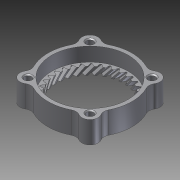
# Autodesk Inventor part: Inner_Helical_Gear_34.5mmOD_3x11.5mmID_4mmH_0.1mmBL_40deg_0.8mmM_33T_CCW_Nema17
Saved by Autodesk Inventor 2015 (Build 190159000, 159)
## iProperties
Created: 2014-08-15
Part Number: Inner_Helical_Gear_34.5mmOD_3x11.5mmID_4mmH_0.1mmBL_40deg_0.8mmM_33T_CCW_Nema17
Material: Generic
Document SubType Name: Modeling
Designer: User
Density: 1 g/cm^3
Appearance: Default
Author: User
Autodesk Inventor part; units mm, degrees
ref_plane "YZ Plane" through (0, 0, 0) normal (1, 0, 0) x (0, 1, 0)
ref_plane "XZ Plane" through (0, 0, 0) normal (0, 1, 0) x (-1, 0, 0)
ref_plane "XY Plane" through (0, 0, 0) normal (0, 0, 1) x (1, 0, 0)
sketch "Sketch1" plane through (0, 0, 0) normal (0, 0, 1) x (1, 0, 0)
  spline S0 degree 3 poles (-1.1058, 16.6253) (-1.0811, 16.7025) (-1.0316, 16.857) (-0.9463, 17.0848) (-0.8539, 17.3098) (-0.7542, 17.5317) (-0.6479, 17.7505) (-0.5354, 17.9662) (-0.4175, 18.1789) (-0.3342, 18.3181) (-0.2926, 18.3877) knots 0 0 0 0 0.124996 0.249995 0.374995 0.499995 0.624996 0.749997 0.874998 1 1 1 1
  spline S1 degree 3 poles (1.1058, 16.6253) (1.0811, 16.7025) (1.0316, 16.857) (0.9463, 17.0848) (0.8539, 17.3098) (0.7542, 17.5317) (0.6479, 17.7505) (0.5354, 17.9662) (0.4175, 18.1789) (0.3342, 18.3181) (0.2926, 18.3877) knots 0 0 0 0 0.124996 0.249995 0.374995 0.499995 0.624996 0.749997 0.874998 1 1 1 1
  circle A0 centre (0, 0) radius 18.39 construction
  circle A1 centre (0, 0) radius 15.5639 construction
  circle A2 centre (0, 0) radius 17.2314 construction
  circle A3 centre (0, 0) radius 16.6621
  circle A4 centre (0, 0) radius 20.118
  arc A5 (0.2926, 18.3877) -> (-0.2926, 18.3877) centre (0, 0) ccw
  point P0 (-1.0298, 16.8563)
  point P1 (-0.9451, 17.0843)
  point P2 (-0.8527, 17.3093)
  point P3 (-0.7531, 17.5312)
  point P4 (-0.6469, 17.75)
  point P5 (-0.5345, 17.9657)
  point P6 (-0.4163, 18.1783)
  point P7 (1.0298, 16.8563)
  point P8 (0.9451, 17.0843)
  point P9 (0.8527, 17.3093)
  point P10 (0.7531, 17.5312)
  point P11 (0.6469, 17.75)
  point P12 (0.5345, 17.9657)
  point P13 (0.4163, 18.1783)
  constraints: 6 centre point, 6 point on circle, 43 other
extrude "Extrusion1" add sketch "Sketch1" against normal blind 4 contours S0 A5 S1 A3 | A4
coil "Coil1" sketch "Sketch1" operation cut axis through (0, 0, -10) along (0, 0, -1) pitch 129.0296 turns 0.031001 hand left contours S0 A5 S1 A3
pattern_circular "Circular Pattern1" count 33 over 360 about axis through (0, 0, 0) along (0, 0, -1) of "Coil1"
sketch "Sketch2" plane through (0, 0, 0) normal (0, 0, 1) x (1, 0, 0)
  line L0 (-15.5, 15.5) -> (15.5, 15.5) construction
  line L1 (15.5, 15.5) -> (15.5, -15.5) construction
  line L2 (15.5, -15.5) -> (-15.5, -15.5) construction
  line L3 (-15.5, -15.5) -> (-15.5, 15.5) construction
  arc A0 (18.9021, 13.3963) -> (13.3963, 18.9021) centre (15.5, 15.5) ccw
  arc A1 (13.3963, -18.9021) -> (18.9021, -13.3963) centre (15.5, -15.5) ccw
  arc A2 (-18.9021, -13.3963) -> (-13.3963, -18.9021) centre (-15.5, -15.5) ccw
  arc A3 (-13.3963, 18.9021) -> (-18.9021, 13.3963) centre (-15.5, 15.5) ccw
  arc A4 (18.7355, -9.4857) -> (18.7355, 9.4857) centre (0, 0) ccw
  arc A5 (-9.4857, -18.7355) -> (9.4857, -18.7355) centre (0, 0) ccw
  arc A6 (9.4857, 18.7355) -> (-9.4857, 18.7355) centre (0, 0) ccw
  arc A7 (-18.7355, 9.4857) -> (-18.7355, -9.4857) centre (0, 0) ccw
  arc A8 (-13.3963, 18.9021) -> (-9.4857, 18.7355) centre (-11.2926, 22.3042) ccw
  arc A9 (9.4857, 18.7355) -> (13.3963, 18.9021) centre (11.2926, 22.3042) ccw
  arc A10 (18.9021, 13.3963) -> (18.7355, 9.4857) centre (22.3042, 11.2926) ccw
  arc A11 (18.7355, -9.4857) -> (18.9021, -13.3963) centre (22.3042, -11.2926) ccw
  arc A12 (13.3963, -18.9021) -> (9.4857, -18.7355) centre (11.2926, -22.3042) ccw
  arc A13 (-9.4857, -18.7355) -> (-13.3963, -18.9021) centre (-11.2926, -22.3042) ccw
  arc A14 (-18.9021, -13.3963) -> (-18.7355, -9.4857) centre (-22.3042, -11.2926) ccw
  arc A15 (-18.7355, 9.4857) -> (-18.9021, 13.3963) centre (-22.3042, 11.2926) ccw
  circle A16 centre (0, 0) radius 20.118 projected
  point P0 (15.5, 0)
  point P1 (0, 15.5)
  dimension "d14" = 31
  dimension "d15" = 31
  dimension "d16" = 8
  dimension "d17" = 8
  dimension "d18" = 8
  dimension "d19" = 8
  dimension "d20" = 21
  dimension "d21" = 21
  dimension "d22" = 21
  dimension "d23" = 21
  dimension "d24" = 4
  constraints: 32 point on circle, 16 centre point, 16 tangent, 8 end point, 7 equal radius, 5 coincident, 2 midpoint, 2 parallel, 1 horizontal, 1 horizontal alignment, 1 perpendicular, 1 vertical alignment
  measures "d14" distance of L0.start L0.end
  measures "d15" distance of L0.end L1.end
  measures "d16" diameter of A0
  measures "d17" diameter of A1
  measures "d18" diameter of A2
  measures "d19" diameter of A3
  measures "d20" radius of A4
  measures "d21" radius of A6
  measures "d22" radius of A7
  measures "d23" radius of A5
  measures "d24" radius of A8
extrude "Extrusion2" add sketch "Sketch2" against normal blind 4
sketch "Sketch3" plane through (0, 0, 0) normal (0, 0, 1) x (1, 0, 0)
  arc A0 (-13.3963, 18.9021) -> (-9.4857, 18.7355) centre (-11.2926, 22.3042) ccw projected
  arc A1 (-13.3963, 18.9021) -> (-18.9021, 13.3963) centre (-15.5, 15.5) ccw projected
  arc A2 (-18.7355, 9.4857) -> (-18.9021, 13.3963) centre (-22.3042, 11.2926) ccw projected
  arc A3 (-18.7355, 9.4857) -> (-18.7355, -9.4857) centre (0, 0) ccw projected
  arc A4 (-18.9021, -13.3963) -> (-18.7355, -9.4857) centre (-22.3042, -11.2926) ccw projected
  arc A5 (-18.9021, -13.3963) -> (-13.3963, -18.9021) centre (-15.5, -15.5) ccw projected
  arc A6 (-9.4857, -18.7355) -> (-13.3963, -18.9021) centre (-11.2926, -22.3042) ccw projected
  arc A7 (-9.4857, -18.7355) -> (9.4857, -18.7355) centre (0, 0) ccw projected
  arc A8 (13.3963, -18.9021) -> (9.4857, -18.7355) centre (11.2926, -22.3042) ccw projected
  arc A9 (13.3963, -18.9021) -> (18.9021, -13.3963) centre (15.5, -15.5) ccw projected
  arc A10 (18.7355, -9.4857) -> (18.9021, -13.3963) centre (22.3042, -11.2926) ccw projected
  arc A11 (18.7355, -9.4857) -> (18.7355, 9.4857) centre (0, 0) ccw projected
  arc A12 (18.9021, 13.3963) -> (18.7355, 9.4857) centre (22.3042, 11.2926) ccw projected
  arc A13 (18.9021, 13.3963) -> (13.3963, 18.9021) centre (15.5, 15.5) ccw projected
  arc A14 (9.4857, 18.7355) -> (13.3963, 18.9021) centre (11.2926, 22.3042) ccw projected
  arc A15 (9.4857, 18.7355) -> (-9.4857, 18.7355) centre (0, 0) ccw projected
  arc A16 (-1.1058, 16.6253) -> (-2.0605, 16.5342) centre (0, 0) ccw projected
  arc A17 (2.0605, 16.5342) -> (1.1058, 16.6253) centre (0, 0) ccw projected
  arc A18 (5.1524, 15.8454) -> (4.2322, 16.1156) centre (0, 0) ccw projected
  arc A19 (8.0581, 14.584) -> (7.2056, 15.0234) centre (0, 0) ccw projected
  arc A20 (10.6725, 12.7954) -> (9.9186, 13.3883) centre (0, 0) ccw projected
  arc A21 (12.9012, 10.5444) -> (12.2731, 11.2692) centre (0, 0) ccw projected
  arc A22 (14.6636, 7.9123) -> (14.184, 8.7429) centre (0, 0) ccw projected
  arc A23 (15.896, 4.9942) -> (15.5823, 5.9005) centre (0, 0) ccw projected
  arc A24 (16.5539, 1.8956) -> (16.4174, 2.8449) centre (0, 0) ccw projected
  arc A25 (16.6135, -1.2715) -> (16.6591, -0.3135) centre (0, 0) ccw projected
  arc A26 (16.0726, -4.3926) -> (16.2987, -3.4606) centre (0, 0) ccw projected
  arc A27 (14.9509, -7.355) -> (15.3493, -6.4826) centre (0, 0) ccw projected
  arc A28 (13.2887, -10.0516) -> (13.845, -9.2703) centre (0, 0) ccw projected
  arc A29 (11.1463, -12.3848) -> (11.8404, -11.723) centre (0, 0) ccw projected
  arc A30 (8.601, -14.2705) -> (9.4079, -13.752) centre (0, 0) ccw projected
  arc A31 (5.7449, -15.6403) -> (6.6353, -15.2839) centre (0, 0) ccw projected
  arc A32 (2.6811, -16.4449) -> (3.6229, -16.2634) centre (0, 0) ccw projected
  arc A33 (-0.4795, -16.6552) -> (0.4795, -16.6552) centre (0, 0) ccw projected
  arc A34 (-3.6229, -16.2634) -> (-2.6811, -16.4449) centre (0, 0) ccw projected
  arc A35 (-6.6353, -15.2839) -> (-5.7449, -15.6403) centre (0, 0) ccw projected
  arc A36 (-9.4079, -13.752) -> (-8.601, -14.2705) centre (0, 0) ccw projected
  arc A37 (-11.8404, -11.723) -> (-11.1463, -12.3848) centre (0, 0) ccw projected
  arc A38 (-13.845, -9.2703) -> (-13.2887, -10.0516) centre (0, 0) ccw projected
  arc A39 (-15.3493, -6.4826) -> (-14.9509, -7.355) centre (0, 0) ccw projected
  arc A40 (-16.2987, -3.4606) -> (-16.0726, -4.3926) centre (0, 0) ccw projected
  arc A41 (-16.6591, -0.3135) -> (-16.6135, -1.2715) centre (0, 0) ccw projected
  arc A42 (-16.4174, 2.8449) -> (-16.5539, 1.8956) centre (0, 0) ccw projected
  arc A43 (-15.5823, 5.9005) -> (-15.896, 4.9942) centre (0, 0) ccw projected
  arc A44 (-14.184, 8.7429) -> (-14.6636, 7.9123) centre (0, 0) ccw projected
  arc A45 (-12.2731, 11.2692) -> (-12.9012, 10.5444) centre (0, 0) ccw projected
  arc A46 (-9.9186, 13.3883) -> (-10.6725, 12.7954) centre (0, 0) ccw projected
  arc A47 (-7.2056, 15.0234) -> (-8.0581, 14.584) centre (0, 0) ccw projected
  arc A48 (-4.2322, 16.1156) -> (-5.1524, 15.8454) centre (0, 0) ccw projected
  circle A49 centre (15.5, 15.5) radius 1.7
  circle A50 centre (-15.5, 15.5) radius 1.7
  circle A51 centre (15.5, -15.5) radius 1.7
  circle A52 centre (-15.5, -15.5) radius 1.7
  dimension "d27" = 3.4
  dimension "d28" = 3.4
  dimension "d29" = 3.4
  dimension "d30" = 3.4
  constraints: 4 centre point, 4 coincident, 1 horizontal alignment, 98 other
  measures "d27" diameter of A49
  measures "d28" diameter of A50
  measures "d29" diameter of A51
  measures "d30" diameter of A52
extrude "Extrusion3" cut sketch "Sketch3" against normal through all contours A49 | A50 | A51 | A52
sketch "Sketch4" plane through (0, 0, 0) normal (0, 0, 1) x (1, 0, 0)
  circle A0 centre (0, 0) radius 19.15
  arc A1 (-18.7355, 9.4857) -> (-18.7355, -9.4857) centre (0, 0) ccw projected
  circle A2 centre (15.5, -15.5) radius 1.7 projected
  circle A3 centre (15.5, 15.5) radius 1.7 projected
  circle A4 centre (-15.5, 15.5) radius 1.7 projected
  circle A5 centre (-15.5, -15.5) radius 1.7 projected
  arc A6 (-13.3963, 18.9021) -> (-9.4857, 18.7355) centre (-11.2926, 22.3042) ccw projected
  arc A7 (-13.3963, 18.9021) -> (-18.9021, 13.3963) centre (-15.5, 15.5) ccw projected
  arc A8 (-18.7355, 9.4857) -> (-18.9021, 13.3963) centre (-22.3042, 11.2926) ccw projected
  arc A9 (-18.7355, 9.4857) -> (-18.7355, -9.4857) centre (0, 0) ccw projected
  arc A10 (-18.9021, -13.3963) -> (-18.7355, -9.4857) centre (-22.3042, -11.2926) ccw projected
  arc A11 (-18.9021, -13.3963) -> (-13.3963, -18.9021) centre (-15.5, -15.5) ccw projected
  arc A12 (-9.4857, -18.7355) -> (-13.3963, -18.9021) centre (-11.2926, -22.3042) ccw projected
  arc A13 (-9.4857, -18.7355) -> (9.4857, -18.7355) centre (0, 0) ccw projected
  arc A14 (13.3963, -18.9021) -> (9.4857, -18.7355) centre (11.2926, -22.3042) ccw projected
  arc A15 (13.3963, -18.9021) -> (18.9021, -13.3963) centre (15.5, -15.5) ccw projected
  arc A16 (18.7355, -9.4857) -> (18.9021, -13.3963) centre (22.3042, -11.2926) ccw projected
  arc A17 (18.7355, -9.4857) -> (18.7355, 9.4857) centre (0, 0) ccw projected
  arc A18 (18.9021, 13.3963) -> (18.7355, 9.4857) centre (22.3042, 11.2926) ccw projected
  arc A19 (18.9021, 13.3963) -> (13.3963, 18.9021) centre (15.5, 15.5) ccw projected
  arc A20 (9.4857, 18.7355) -> (13.3963, 18.9021) centre (11.2926, 22.3042) ccw projected
  arc A21 (9.4857, 18.7355) -> (-9.4857, 18.7355) centre (0, 0) ccw projected
  arc A22 (-1.1058, 16.6253) -> (-2.0605, 16.5342) centre (0, 0) ccw projected
  arc A23 (2.0605, 16.5342) -> (1.1058, 16.6253) centre (0, 0) ccw projected
  arc A24 (5.1524, 15.8454) -> (4.2322, 16.1156) centre (0, 0) ccw projected
  arc A25 (8.0581, 14.584) -> (7.2056, 15.0234) centre (0, 0) ccw projected
  arc A26 (10.6725, 12.7954) -> (9.9186, 13.3883) centre (0, 0) ccw projected
  arc A27 (12.9012, 10.5444) -> (12.2731, 11.2692) centre (0, 0) ccw projected
  arc A28 (14.6636, 7.9123) -> (14.184, 8.7429) centre (0, 0) ccw projected
  arc A29 (15.896, 4.9942) -> (15.5823, 5.9005) centre (0, 0) ccw projected
  arc A30 (16.5539, 1.8956) -> (16.4174, 2.8449) centre (0, 0) ccw projected
  arc A31 (16.6135, -1.2715) -> (16.6591, -0.3135) centre (0, 0) ccw projected
  arc A32 (16.0726, -4.3926) -> (16.2987, -3.4606) centre (0, 0) ccw projected
  arc A33 (14.9509, -7.355) -> (15.3493, -6.4826) centre (0, 0) ccw projected
  arc A34 (13.2887, -10.0516) -> (13.845, -9.2703) centre (0, 0) ccw projected
  arc A35 (11.1463, -12.3848) -> (11.8404, -11.723) centre (0, 0) ccw projected
  arc A36 (8.601, -14.2705) -> (9.4079, -13.752) centre (0, 0) ccw projected
  arc A37 (5.7449, -15.6403) -> (6.6353, -15.2839) centre (0, 0) ccw projected
  arc A38 (2.6811, -16.4449) -> (3.6229, -16.2634) centre (0, 0) ccw projected
  arc A39 (-0.4795, -16.6552) -> (0.4795, -16.6552) centre (0, 0) ccw projected
  arc A40 (-3.6229, -16.2634) -> (-2.6811, -16.4449) centre (0, 0) ccw projected
  arc A41 (-6.6353, -15.2839) -> (-5.7449, -15.6403) centre (0, 0) ccw projected
  arc A42 (-9.4079, -13.752) -> (-8.601, -14.2705) centre (0, 0) ccw projected
  arc A43 (-11.8404, -11.723) -> (-11.1463, -12.3848) centre (0, 0) ccw projected
  arc A44 (-13.845, -9.2703) -> (-13.2887, -10.0516) centre (0, 0) ccw projected
  arc A45 (-15.3493, -6.4826) -> (-14.9509, -7.355) centre (0, 0) ccw projected
  arc A46 (-16.2987, -3.4606) -> (-16.0726, -4.3926) centre (0, 0) ccw projected
  arc A47 (-16.6591, -0.3135) -> (-16.6135, -1.2715) centre (0, 0) ccw projected
  arc A48 (-16.4174, 2.8449) -> (-16.5539, 1.8956) centre (0, 0) ccw projected
  arc A49 (-15.5823, 5.9005) -> (-15.896, 4.9942) centre (0, 0) ccw projected
  arc A50 (-14.184, 8.7429) -> (-14.6636, 7.9123) centre (0, 0) ccw projected
  arc A51 (-12.2731, 11.2692) -> (-12.9012, 10.5444) centre (0, 0) ccw projected
  arc A52 (-9.9186, 13.3883) -> (-10.6725, 12.7954) centre (0, 0) ccw projected
  arc A53 (-7.2056, 15.0234) -> (-8.0581, 14.584) centre (0, 0) ccw projected
  arc A54 (-4.2322, 16.1156) -> (-5.1524, 15.8454) centre (0, 0) ccw projected
  dimension "d36" = 38.3
  constraints: 1 centre point, 1 coincident, 1 horizontal alignment, 98 other
  measures "d36" diameter of A0
extrude "Extrusion4" add sketch "Sketch4" along normal blind 7
chamfer "Chamfer1" distance 0.5 angle 45 8 edges at (13.8, -15.5, -4) (13.8, 15.5, -4) (-17.2, 15.5, -4) (-17.2, -15.5, -4) (-17.2, -15.5, 7) (-17.2, 15.5, 7) (13.8, 15.5, 7) (13.8, -15.5, 7)
equation "\"d0\" = FaceWidth"
equation "\"Module\" = 0.8"
equation "\"PressureAngle\" = 20deg"
equation "\"UnitProfileClearance\" = 0.25"
equation "\"UnitRoundRadius\" = 0.35"
equation "\"HeadDiameter\" = 33.32412"
equation "\"RootDiameter\" = 36.78002"
equation "\"BaseDiameter\" = 31.12787"
equation "\"PitchDiameter\" = 34.46275"
equation "\"FaceWidth\" = 4"
equation "\"HelixAngle\" = 40deg"
equation "\"UnitCorrection\" = 0.015557"
equation "\"UnitAddendumModification\" = 0.272795"
equation "\"CircularPitch\" = 3.28085"
equation "\"UnitBacklashShift\" = 0.182738"
equation "\"TotalToolShift\" = 0.15864"
body "Solid1"
